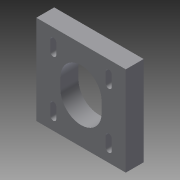
# Autodesk Inventor part: nema17gen
Saved by Autodesk Inventor 2014 (Build 180170000, 170)
## iProperties
Created: 2014-07-13
Part Number: nema17gen
Material: Generic
Document SubType Name: Modeling
Designer: cruiser
Density: 1 g/cm^3
Appearance: Default
Author: cruiser
Autodesk Inventor part; units mm, degrees
ref_plane "YZ Plane" through (0, 0, 0) normal (1, 0, 0) x (0, 1, 0)
ref_plane "XZ Plane" through (0, 0, 0) normal (0, 1, 0) x (-1, 0, 0)
ref_plane "XY Plane" through (0, 0, 0) normal (0, 0, 1) x (1, 0, 0)
sketch "Sketch1" plane through (0, 0, 0) normal (0, 1, 0) x (-1, 0, 0)
  line L0 (25, -25) -> (-25, -25)
  line L1 (-25, -25) -> (-25, 25)
  line L2 (-25, 25) -> (25, 25)
  line L3 (25, 25) -> (25, -25)
  line L4 (25, -25) -> (-25, 25) construction
  line L5 (-25, -25) -> (25, 25) construction
  point P0 (0, 0)
  dimension "d0" = 50
  dimension "d1" = 50
  constraints: 12 end point, 2 midpoint, 2 parallel, 1 horizontal, 1 perpendicular
  measures "d0" distance of L1.end L2.end
  measures "d1" distance of L0.end L1.end
extrude "Extrusion1" add sketch "Sketch1" along normal blind 10
sketch "Sketch5" plane through (0, 0, 0) normal (0, -1, 0) x (1, 0, 0)
  line L0 (15.5, -15.5) -> (-15.5, -15.5)
  line L1 (-15.5, -15.5) -> (-15.5, 15.5)
  line L2 (-15.5, 15.5) -> (15.5, 15.5)
  line L3 (15.5, 15.5) -> (15.5, -15.5)
  line L4 (15.5, -15.5) -> (-15.5, 15.5) construction
  line L5 (-15.5, -15.5) -> (15.5, 15.5) construction
  line L6 (0, -3) -> (0, 3) construction
  line L7 (11.5, -3) -> (11.5, 3)
  line L8 (-11.5, 3) -> (-11.5, -3)
  arc A0 (-11.5, -3) -> (11.5, -3) centre (0, -3) ccw
  arc A1 (11.5, 3) -> (-11.5, 3) centre (0, 3) ccw
  line L9 (-15.5, 12.5) -> (-15.5, 18.5) construction
  line L10 (-13.85, 12.5) -> (-13.85, 18.5)
  line L11 (-17.15, 18.5) -> (-17.15, 12.5)
  arc A2 (-17.15, 12.5) -> (-13.85, 12.5) centre (-15.5, 12.5) ccw
  arc A3 (-13.85, 18.5) -> (-17.15, 18.5) centre (-15.5, 18.5) ccw
  line L12 (15.5, 12.5) -> (15.5, 18.5) construction
  line L13 (17.15, 12.5) -> (17.15, 18.5)
  line L14 (13.85, 18.5) -> (13.85, 12.5)
  arc A4 (13.85, 12.5) -> (17.15, 12.5) centre (15.5, 12.5) ccw
  arc A5 (17.15, 18.5) -> (13.85, 18.5) centre (15.5, 18.5) ccw
  line L15 (-15.5, -18.5) -> (-15.5, -12.5) construction
  line L16 (-13.85, -18.5) -> (-13.85, -12.5)
  line L17 (-17.15, -12.5) -> (-17.15, -18.5)
  arc A6 (-17.15, -18.5) -> (-13.85, -18.5) centre (-15.5, -18.5) ccw
  arc A7 (-13.85, -12.5) -> (-17.15, -12.5) centre (-15.5, -12.5) ccw
  line L18 (15.5, -18.5) -> (15.5, -12.5) construction
  line L19 (17.15, -18.5) -> (17.15, -12.5)
  line L20 (13.85, -12.5) -> (13.85, -18.5)
  arc A8 (13.85, -18.5) -> (17.15, -18.5) centre (15.5, -18.5) ccw
  arc A9 (17.15, -12.5) -> (13.85, -12.5) centre (15.5, -12.5) ccw
  point P0 (0, 0)
  dimension "d39" = 31
  dimension "d40" = 31
  dimension "d41" = 3
  dimension "d42" = 23
  dimension "d43" = 3
  dimension "d44" = 3.3
  dimension "d45" = 3
  dimension "d46" = 3.3
  dimension "d47" = 3
  dimension "d48" = 3.3
  dimension "d49" = 3
  dimension "d50" = 3.3
  constraints: 52 end point, 20 point on circle, 20 tangent, 10 centre point, 10 parallel, 7 midpoint, 2 point on line, 1 horizontal, 1 perpendicular
  measures "d39" distance of L1.end L2.end
  measures "d40" distance of L0.end L1.end
  measures "d41" distance of point (0, 0) L6.end
  measures "d42" diameter of A1
  measures "d43" distance of L1.end L9.end
  measures "d44" diameter of A3
  measures "d45" distance of L2.end L12.end
  measures "d46" diameter of A5
  measures "d47" distance of L0.end L15.end
  measures "d48" diameter of A7
  measures "d49" distance of L0.start L18.end
  measures "d50" diameter of A9
extrude "Extrusion5" cut sketch "Sketch5" against normal up to next contours L3 A9 L19 A8 L20 L0 | L0 L20 A9 L3 | L16 A6 L17 A7 L1 L0 | L0 L1 A7 L16 | A4 L14 L2 L3 | L3 L2 L14 A5 L13 A4 | A2 L11 A3 L10 L2 L1 | L1 L2 L10 A2 | A0 L8 A1 L7
sketch "Sketch4" plane through (0, 0, 0) normal (0, -1, 0) x (1, 0, 0)
  line L0 (25, -25) -> (25, 25) projected
  line L1 (0, -3) -> (0, 3) construction
  line L2 (11.5, -3) -> (11.5, 3)
  line L3 (-11.5, 3) -> (-11.5, -3)
  arc A0 (-11.5, -3) -> (11.5, -3) centre (0, -3) ccw
  arc A1 (11.5, 3) -> (-11.5, 3) centre (0, 3) ccw
  line L4 (15.5, -15.5) -> (-15.5, -15.5)
  line L5 (-15.5, -15.5) -> (-15.5, 15.5)
  line L6 (-15.5, 15.5) -> (15.5, 15.5)
  line L7 (15.5, 15.5) -> (15.5, -15.5)
  line L8 (15.5, -15.5) -> (-15.5, 15.5) construction
  line L9 (-15.5, -15.5) -> (15.5, 15.5) construction
  line L10 (-15.5, 12.5) -> (-15.5, 18.5) construction
  line L11 (-13.85, 12.5) -> (-13.85, 18.5)
  line L12 (-17.15, 18.5) -> (-17.15, 12.5)
  arc A2 (-17.15, 12.5) -> (-13.85, 12.5) centre (-15.5, 12.5) ccw
  arc A3 (-13.85, 18.5) -> (-17.15, 18.5) centre (-15.5, 18.5) ccw
  line L13 (15.5, 12.5) -> (15.5, 18.5) construction
  line L14 (17.15, 12.5) -> (17.15, 18.5)
  line L15 (13.85, 18.5) -> (13.85, 12.5)
  arc A4 (13.85, 12.5) -> (17.15, 12.5) centre (15.5, 12.5) ccw
  arc A5 (17.15, 18.5) -> (13.85, 18.5) centre (15.5, 18.5) ccw
  line L16 (-15.5, -18.5) -> (-15.5, -12.5) construction
  line L17 (-13.85, -18.5) -> (-13.85, -12.5)
  line L18 (-17.15, -12.5) -> (-17.15, -18.5)
  arc A6 (-17.15, -18.5) -> (-13.85, -18.5) centre (-15.5, -18.5) ccw
  arc A7 (-13.85, -12.5) -> (-17.15, -12.5) centre (-15.5, -12.5) ccw
  line L19 (15.5, -18.5) -> (15.5, -12.5) construction
  line L20 (17.15, -18.5) -> (17.15, -12.5)
  line L21 (13.85, -12.5) -> (13.85, -18.5)
  arc A8 (13.85, -18.5) -> (17.15, -18.5) centre (15.5, -18.5) ccw
  arc A9 (17.15, -12.5) -> (13.85, -12.5) centre (15.5, -12.5) ccw
  line L22 (25, -25) -> (-25, -25)
  line L23 (-25, -25) -> (-25, 25)
  line L24 (-25, 25) -> (25, 25)
  line L25 (25, 25) -> (25, -25)
  line L26 (25, -25) -> (-25, 25) construction
  line L27 (-25, -25) -> (25, 25) construction
  line L28 (0, 0) -> (0, 25)
  line L29 (0, 0) -> (-25, 0)
  line L30 (0, 0) -> (25, 0)
  line L31 (0, 0) -> (0, -25)
  dimension "d25" = 3
  dimension "d26" = 23
  dimension "d27" = 31
  dimension "d28" = 31
  dimension "d29" = 3
  dimension "d30" = 3.3
  dimension "d31" = 3
  dimension "d32" = 3.3
  dimension "d33" = 3
  dimension "d34" = 3.3
  dimension "d35" = 3
  dimension "d36" = 3.3
  constraints: 72 end point, 20 point on circle, 20 tangent, 15 midpoint, 11 parallel, 10 centre point, 3 perpendicular, 2 horizontal, 2 point on line
  measures "d25" distance of L28.start L1.end
  measures "d26" distance between parallel lines of L2 L3
  measures "d27" distance of L5.end L6.end
  measures "d28" distance of L4.end L5.end
  measures "d29" distance of L5.end L10.end
  measures "d30" diameter of A3
  measures "d31" distance of L6.end L13.end
  measures "d32" diameter of A5
  measures "d33" distance of L4.end L16.end
  measures "d34" diameter of A7
  measures "d35" distance of L4.start L19.end
  measures "d36" diameter of A9
equation "\"d41\" = slot"
equation "\"d43\" = slot"
equation "\"d44\" = mount_hole_d"
equation "\"d45\" = slot"
equation "\"d46\" = mount_hole_d"
equation "\"d47\" = slot"
equation "\"d48\" = mount_hole_d"
equation "\"d49\" = slot"
equation "\"d50\" = mount_hole_d"
equation "\"d25\" = slot"
equation "\"d29\" = slot"
equation "\"d31\" = slot"
equation "\"d33\" = slot"
equation "\"d35\" = slot"
equation "\"slot\" = 3"
equation "\"mount_hole_d\" = 3.3"
body "Solid1"
